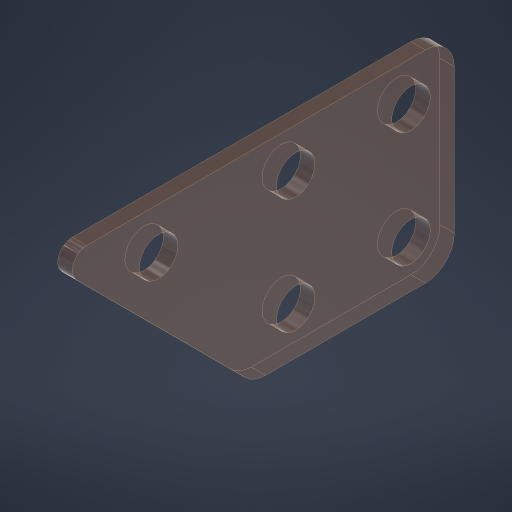
# Autodesk Inventor part: sled
Saved by Autodesk Inventor 2024 (Build 280153000, 153)
## iProperties
Created: 2023-08-09
Part Number: sled
Material: Polycarbonate, Smoke
Document SubType Name: Modeling
Designer: macbook
Density: 1.2 g/cm^3
Appearance: Polycarbonate - Smoked
Author: macbook
Autodesk Inventor part; units mm, degrees
ref_plane "YZ Plane" through (0, 0, 0) normal (1, 0, 0) x (0, 1, 0)
ref_plane "XZ Plane" through (0, 0, 0) normal (0, 1, 0) x (-1, 0, 0)
ref_plane "XY Plane" through (0, 0, 0) normal (0, 0, 1) x (1, 0, 0)
sketch "Sketch1" plane through (0, 0, 0) normal (1, 0, 0) x (0, 1, 0)
  arc A0 (0, -19.05) -> (3.175, -22.225) centre (3.175, -19.05) ccw
  arc A1 (19.05, -22.225) -> (22.225, -19.05) centre (19.05, -19.05) ccw
  line L0 (0, -1.4407) -> (0, -19.05)
  line L1 (0.9299, 0.8044) -> (19.515, 19.3894)
  line L2 (22.225, 18.2669) -> (22.225, -19.05)
  line L3 (19.05, -22.225) -> (3.175, -22.225)
  arc A2 (22.225, 18.2669) -> (19.515, 19.3894) centre (20.6375, 18.2669) ccw
  arc A3 (0.9299, 0.8044) -> (0, -1.4407) centre (3.175, -1.4407) ccw
  point P0 (0, -22.225)
  point P1 (22.225, -22.225)
  dimension "d1" = 22.225
  dimension "d6" = 3.175
  dimension "d46" = 1.5875
  dimension "d47" = 3.175
  constraints: 8 end point, 8 point on circle, 6 tangent, 4 centre point, 2 vertical, 1 equal radius, 1 horizontal
  measures "d1" distance of point (0, -22.225) point (22.225, -22.225)
  measures "d6" radius of A0
  measures "d46" radius of A2
  measures "d47" radius of A3
extrude "Extrusion1" add sketch "Sketch1" along normal blind 1.5875
sketch "Sketch2" plane through (1.5875, 0, 0) normal (1, 0, 0) x (0, 0, -1)
  line L0 (22.225, 3.175) -> (22.225, 19.05) projected
  line L1 (0, 11.1125) -> (4.7625, 11.1125)
  line L2 (4.7625, 11.1125) -> (17.4625, 11.1125)
  line L3 (17.4625, 11.1125) -> (22.225, 11.1125)
  line L4 (4.7625, 11.1125) -> (4.7625, 17.4625)
  line L5 (17.4625, 17.4625) -> (17.4625, 4.7625)
  line L6 (4.7625, 4.7625) -> (4.7625, 11.1125)
  line L7 (4.7625, 17.4625) -> (-17.3369, 17.4625)
  line L8 (-19.3894, 19.515) -> (-0.8044, 0.9299) projected
  line L9 (-17.3369, 17.4625) -> (-13.9604, 20.8391)
  line L10 (-17.3369, 17.4625) -> (-12.5617, 17.4625) construction
  line L11 (-13.9604, 20.8391) -> (-6.7223, 13.601)
  line L12 (-13.9604, 20.8391) -> (-3.7242, 20.8391) construction
  point P0 (0, 0)
  point P1 (-10.3413, 17.22)
  dimension "d13" = 4.7625
  dimension "d14" = 12.7
  dimension "d15" = 6.35
  dimension "d16" = 12.7
  dimension "d49" = 4.7752
  dimension "d50" = 45
  dimension "d51" = 10.2362
  dimension "d52" = 45
  constraints: 22 end point, 4 coincident, 4 horizontal, 2 equal length, 2 midpoint, 2 vertical, 1 perpendicular, 1 point on line
  measures "d13" distance of L1.start L1.end
  measures "d14" distance of L1.end L2.end
  measures "d15" distance of L1.end L4.end
  measures "d16" distance of L5.start L5.end
  measures "d49" distance of L7.end L9.end
  measures "d50" angle of L10 L9
  measures "d51" distance of L9.end L11.end
  measures "d52" angle of L11 L12
hole "Hole1" at (1.5875, 17.4625, -4.7625) at (1.5875, 4.7625, -4.7625) at (1.5875, 17.22, 10.3413) at (1.5875, 17.4625, -17.4625) at (1.5875, 4.7625, -17.4625) direction (-1, 0, 0) diameter 4.2418 end through all
sketch "Sketch3" plane through (1.5875, 0, 0) normal (1, 0, 0) x (0, 0, -1)
  line L0 (1.4407, 0) -> (19.05, 0) projected
  line L1 (12.4554, 0) -> (12.4554, 22.225)
  line L2 (19.05, 22.225) -> (-18.2669, 22.225) projected
  point P0 (0, 0)
  constraints: 2 end point, 2 point on line, 1 vertical
split "Split1" [suppressed]
body "Solid1"
